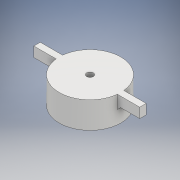
# Autodesk Inventor part: RescueKitThrow_bottom
Saved by Autodesk Inventor 2018.3 (Build 223284000, 284)
## iProperties
Created: 2019-02-10
Part Number: RescueKitThrow_bottom
Material: ABS プラスチック
Document SubType Name: Modeling
Designer: shun2
Density: 1.06 g/cm^3
Appearance: 滑らか - 白
Author: shun2
Autodesk Inventor part; units mm, degrees
ref_plane "YZ Plane" through (0, 0, 0) normal (1, 0, 0) x (0, 1, 0)
ref_plane "XZ Plane" through (0, 0, 0) normal (0, 1, 0) x (-1, 0, 0)
ref_plane "XY Plane" through (0, 0, 0) normal (0, 0, 1) x (1, 0, 0)
sketch "スケッチ1" plane through (0, 0, 0) normal (0, 0, 1) x (1, 0, 0)
  line L0 (-16, 0.9789) -> (-9.2483, 0.9789)
  line L1 (-9.2483, -0.9789) -> (-16, -0.9789)
  line L2 (-16, -0.9789) -> (-16, 0.9789)
  line L3 (16, 0.9789) -> (9.2483, 0.9789)
  line L4 (9.2483, -0.9789) -> (16, -0.9789)
  arc A0 (9.2483, 0.9789) -> (-9.2483, 0.9789) centre (0, 0) ccw
  arc A1 (-9.2483, -0.9789) -> (9.2483, -0.9789) centre (0, 0) ccw
  line L5 (16, -0.9789) -> (16, 0.9789)
  circle A2 centre (0, 0) radius 1
  dimension "d3" = 2
  dimension "d6" = 16
  dimension "d7" = 16
  dimension "d17" = 9.3
  dimension "d18" = 9.3
  constraints: 12 end point, 4 point on circle, 3 centre point, 2 coincident, 2 horizontal, 2 parallel, 1 vertical
  measures "d3" diameter of A2
  measures "d6" distance from line of L2 point (0, 0)
  measures "d7" distance from line of L5 point (0, 0)
  measures "d17" radius of A0
  measures "d18" radius of A1
extrude "押し出し1" add sketch "スケッチ1" along normal blind 3
sketch "スケッチ2" plane through (0, 0, 0) normal (0, 0, -1) x (-1, 0, 0)
  circle A0 centre (0, 0) radius 5
  arc A1 (9.2483, 0.9789) -> (-9.2483, 0.9789) centre (0, 0) ccw projected
  line L0 (9.2483, -0.9789) -> (16, -0.9789) projected
  line L1 (-16, -0.9789) -> (-16, 0.9789) projected
  circle A2 centre (0, 0) radius 9.3
  dimension "d8" = 10
  constraints: 2 centre point, 2 coincident, 1 concentric
  measures "d8" diameter of A0
extrude "押し出し2" add sketch "スケッチ2" along normal blind 5
chamfer "面取り1" distance 1 angle 45 1 edges at (5, 0, 0)
chamfer "面取り2" distance 1 angle 45 3 edges at (9.3, 0, 0) (-9.2871, 0.4902, 0) (-9.2871, -0.4902, 0)
